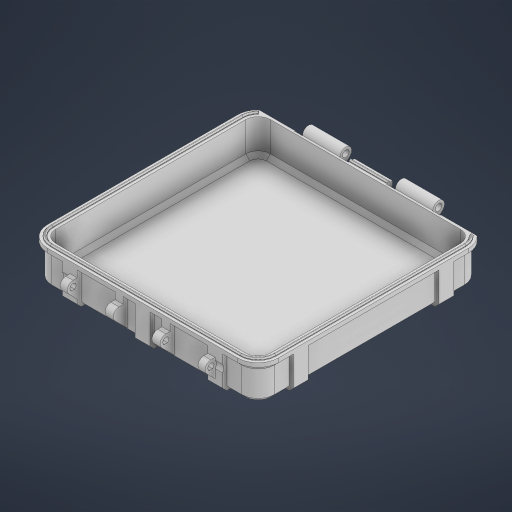
# Autodesk Inventor part: sumec_box-lid
Saved by Autodesk Inventor 2024 (Build 280153000, 153)
## iProperties
Created: 2024-03-05
Part Number: sumec_box-lid
Material: Všeobecné
Document SubType Name: Modeling
Designer: Simak
Density: 1 g/cm^3
Appearance: Výchozí
Author: Simak
Autodesk Inventor part; units mm, degrees
ref_plane "YZ Plane" through (0, 0, 0) normal (1, 0, 0) x (0, 1, 0)
ref_plane "XZ Plane" through (0, 0, 0) normal (0, 1, 0) x (-1, 0, 0)
sketch "velikost" plane through (0, 0, 0) normal (0, 1, 0) x (-1, 0, 0)
  line L0 (54.5, -54.5) -> (-54.5, -54.5)
  line L1 (-54.5, -54.5) -> (-54.5, 54.5)
  line L2 (-54.5, 54.5) -> (54.5, 54.5)
  line L3 (54.5, 54.5) -> (54.5, -54.5)
  line L4 (54.5, -54.5) -> (0, 0) construction
  line L5 (0, 0) -> (-54.5, -54.5) construction
  line L6 (0, 0) -> (-54.5, 54.5) construction
  dimension "d0" = 109
  dimension "d1" = 109
  constraints: 14 end point, 2 equal length, 2 parallel, 1 horizontal, 1 perpendicular
  measures "d0" distance of L0.start L0.end
  measures "d1" distance of L0.end L1.end
extrude "vyska" add sketch "velikost" along normal blind 18.5
fillet "Zaobleni_rohu" radius 8 4 edges at (-54.5, 9.25, 54.5) (54.5, 9.25, 54.5) (54.5, 9.25, -54.5) (-54.5, 9.25, -54.5)
shell "tloustka_sten" thickness 2 removed faces 1 at (15.5, 18.5, -12.8333)
sketch "vyztuhy-velikost" plane through (0, 18.5, 0) normal (0, 1, 0) x (1, 0, 0)
  arc A0 (-46.5, 52.5) -> (-52.5, 46.5) centre (-46.5, 46.5) ccw projected
  line L0 (-46.5, 52.5) -> (46.5, 52.5) projected
  arc A1 (52.5, 46.5) -> (46.5, 52.5) centre (46.5, 46.5) ccw projected
  line L1 (52.5, 46.5) -> (52.5, -46.5) projected
  arc A2 (46.5, -52.5) -> (52.5, -46.5) centre (46.5, -46.5) ccw projected
  line L2 (46.5, -52.5) -> (-46.5, -52.5) projected
  arc A3 (-52.5, -46.5) -> (-46.5, -52.5) centre (-46.5, -46.5) ccw projected
  line L3 (-52.5, -46.5) -> (-52.5, 46.5) projected
  arc A4 (-46.5, 54.5) -> (-54.5, 46.5) centre (-46.5, 46.5) ccw projected
  line L4 (-54.5, 46.5) -> (-54.5, -46.5) projected
  arc A5 (-54.5, -46.5) -> (-46.5, -54.5) centre (-46.5, -46.5) ccw projected
  line L5 (-46.5, -54.5) -> (46.5, -54.5) projected
  arc A6 (46.5, -54.5) -> (54.5, -46.5) centre (46.5, -46.5) ccw projected
  line L6 (54.5, -46.5) -> (54.5, 46.5) projected
  arc A7 (54.5, 46.5) -> (46.5, 54.5) centre (46.5, 46.5) ccw projected
  line L7 (46.5, 54.5) -> (-46.5, 54.5) projected
  line L8 (-39.2333, 54.5) -> (-39.2333, 56.5)
  line L9 (-39.2333, 56.5) -> (-31.9667, 56.5)
  line L10 (-31.9667, 56.5) -> (-31.9667, 54.5)
  line L11 (-3.6333, 54.5) -> (-3.6333, 56.5)
  line L12 (-3.6333, 56.5) -> (3.6333, 56.5)
  line L13 (3.6333, 56.5) -> (3.6333, 54.5)
  line L14 (31.9667, 54.5) -> (31.9667, 56.5)
  line L15 (31.9667, 56.5) -> (39.2333, 56.5)
  line L16 (39.2333, 56.5) -> (39.2333, 54.5)
  line L17 (46.5, 54.5) -> (-46.5, 54.5) projected
  line L18 (-3.6333, 56.5) -> (0, 54.5) construction
  line L19 (3.6333, 56.5) -> (0, 54.5) construction
  line L20 (-31.9667, 56.5) -> (-3.6333, 56.5) construction
  line L21 (3.6333, 56.5) -> (31.9667, 56.5) construction
  line L22 (-39.2333, 56.5) -> (-46.5, 56.5) construction
  line L23 (-46.5, 56.5) -> (-46.5, 54.5) construction
  line L24 (-52.5, 0) -> (52.5, 0)
  line L25 (0, 52.5) -> (0, -52.5)
  line L26 (46.5, -52.5) -> (-46.5, -52.5) projected
  line L27 (-54.5, -39.2333) -> (-56.5, -39.2333)
  line L28 (-56.5, -39.2333) -> (-56.5, -31.9667)
  line L29 (-56.5, -31.9667) -> (-54.5, -31.9667)
  line L30 (-54.5, 31.9667) -> (-56.5, 31.9667)
  line L31 (-56.5, 31.9667) -> (-56.5, 39.2333)
  line L32 (-56.5, 39.2333) -> (-54.5, 39.2333)
  line L33 (-56.5, -31.9667) -> (-56.5, 31.9667) construction
  line L34 (-56.5, -39.2333) -> (-56.5, -46.5) construction
  line L35 (-56.5, -46.5) -> (-54.5, -46.5) construction
  line L36 (-54.5, 46.5) -> (-54.5, -46.5) projected
  line L37 (-56.5, 39.2333) -> (-56.5, 46.5) construction
  line L38 (-56.5, 46.5) -> (-54.5, 46.5) construction
  line L39 (-54.5, 0) -> (-56.5, 31.9667) construction
  line L40 (-54.5, 0) -> (-56.5, -31.9667) construction
  line L41 (-39.2333, -54.5) -> (-39.2333, -56.5)
  line L42 (-39.2333, -56.5) -> (-31.9667, -56.5)
  line L43 (-31.9667, -56.5) -> (-31.9667, -54.5)
  line L44 (-3.6333, -54.5) -> (-3.6333, -56.5)
  line L45 (-3.6333, -56.5) -> (3.6333, -56.5)
  line L46 (3.6333, -56.5) -> (3.6333, -54.5)
  line L47 (31.9667, -54.5) -> (31.9667, -56.5)
  line L48 (31.9667, -56.5) -> (39.2333, -56.5)
  line L49 (39.2333, -56.5) -> (39.2333, -54.5)
  line L50 (46.5, -54.5) -> (-46.5, -54.5)
  line L51 (-3.6333, -56.5) -> (0, -54.5) construction
  line L52 (3.6333, -56.5) -> (0, -54.5) construction
  line L53 (-31.9667, -56.5) -> (-3.6333, -56.5) construction
  line L54 (3.6333, -56.5) -> (31.9667, -56.5) construction
  line L55 (-39.2333, -56.5) -> (-46.5, -56.5) construction
  line L56 (-46.5, -56.5) -> (-46.5, -54.5) construction
  line L57 (54.5, 46.5) -> (54.5, -46.5)
  line L58 (56.5, -31.9667) -> (56.5, 31.9667) construction
  line L59 (54.5, -39.2333) -> (56.5, -39.2333)
  line L60 (56.5, -39.2333) -> (56.5, -46.5) construction
  line L61 (56.5, -31.9667) -> (54.5, -31.9667)
  line L62 (56.5, -46.5) -> (54.5, -46.5) construction
  line L63 (56.5, -39.2333) -> (56.5, -31.9667)
  line L64 (56.5, 31.9667) -> (56.5, 39.2333)
  line L65 (56.5, 39.2333) -> (54.5, 39.2333)
  line L66 (54.5, 31.9667) -> (56.5, 31.9667)
  line L67 (54.5, 46.5) -> (54.5, -46.5)
  line L68 (56.5, 39.2333) -> (56.5, 46.5) construction
  line L69 (56.5, 46.5) -> (54.5, 46.5) construction
  line L70 (54.5, 0) -> (56.5, 31.9667) construction
  line L71 (54.5, 0) -> (56.5, -31.9667) construction
  point P0 (0, 0)
  point P1 (54.5, 39.2333)
  point P2 (54.5, 31.9667)
  point P3 (54.5, -31.9667)
  point P4 (39.2333, -54.5)
  point P5 (31.9667, -54.5)
  point P6 (3.6333, -54.5)
  point P7 (-3.6333, -54.5)
  point P8 (-31.9667, -54.5)
  point P9 (-39.2333, -54.5)
  point P10 (-54.5, -31.9667)
  point P11 (-54.5, 31.9667)
  point P12 (-54.5, 39.2333)
  dimension "d6" = 2
  dimension "d7" = 7.2667
  dimension "d8" = 2
  constraints: 120 end point, 25 symmetric about line, 20 point on line, 14 equal length, 11 perpendicular, 5 midpoint, 5 vertical, 2 horizontal, 5 other
  measures "d6" distance of L9.end L10.end
  measures "d7" distance of L11.end L12.end
  measures "d8" distance of L33.start L29.end
extrude "vyztuhy" add sketch "vyztuhy-velikost" against normal up to surface (18.5 mm away) contours L8 L9 L10 L7 | L4 L30 L31 L32 | L11 L12 L13 L7 | L4 L27 L28 L29 | L14 L15 L16 L7 | L5 L43 L42 L41 | L65 L64 L66 L6 | L5 L46 L45 L44 | L61 L63 L59 L6 | L5 L49 L48 L47
chamfer "Zkoseni_spodku" distance 2 angle 45 36 edges at (-17.8, 0, 54.5) (17.8, 0, 54.5) (0, 0, 56.5) (35.6, 0, 56.5) (42.8667, 0, 54.5) (52.1569, 0, 52.1569) (54.5, 0, 42.8667) (56.5, 0, 35.6) (54.5, 0, 0) (56.5, 0, -35.6) (52.1569, 0, -52.1569) (42.8667, 0, -54.5) (54.5, 0, -42.8667) (35.6, 0, -56.5) (17.8, 0, -54.5) (0, 0, -56.5) (-17.8, 0, -54.5) (-35.6, 0, -56.5) (-42.8667, 0, -54.5) (-52.1569, 0, -52.1569) (-54.5, 0, -42.8667) (-56.5, 0, -35.6) (-54.5, 0, 0) (-56.5, 0, 35.6) (-54.5, 0, 42.8667) (-52.1569, 0, 52.1569) (-42.8667, 0, 54.5) (-35.6, 0, 56.5) (-52.5, 2, 0) (-50.7426, 2, 50.7426) (0, 2, 52.5) (50.7426, 2, 50.7426) (52.5, 2, 0) (50.7426, 2, -50.7426) (0, 2, -52.5) (-50.7426, 2, -50.7426)
sketch "Náčrt4" plane through (39.2333, 18.5, -54.5) normal (1, 0, 0) x (0, 0, -1)
  line L0 (-2, 0) -> (-2, -14.5) projected
  line L1 (2, 0) -> (2, -16.5) projected
  line L2 (-8, 0) -> (0, 0) projected
  line L3 (-0.7, 0) -> (-0.7, 0.3)
  line L4 (-0.7, 0.3) -> (0.7, 0.3)
  line L5 (0.7, 0.3) -> (0.7, 0)
  line L6 (-0.7, 0.3) -> (-2, 0.3) construction
  line L7 (0.7, 0.3) -> (2, 0.3) construction
  line L8 (2, 0) -> (0, 0) projected
  line L9 (2, -4) -> (-2, -4)
  line L10 (-0.6, 0.3) -> (-0.1631, 0.9157)
  arc A0 (0.1631, 0.9157) -> (-0.1631, 0.9157) centre (0, 0.8) ccw
  line L11 (0.1631, 0.9157) -> (0.6, 0.3)
  point P0 (-54.5, -18.5)
  point P1 (0, 0.3)
  point P2 (0, 1)
  dimension "d16" = 1.4
  dimension "d71" = 4
  dimension "d72" = 0.3
  dimension "d75" = 1
  dimension "d76" = 0.2
  dimension "d77" = 0.6
  constraints: 16 end point, 9 point on line, 5 perpendicular, 3 point on circle, 3 vertical alignment, 2 equal length, 2 tangent, 1 centre point, 1 midpoint
  measures "d16" distance of L3.end L4.end
  measures "d71" distance between parallel lines of L9 L8
  measures "d72" distance between parallel lines of L8 L4
  measures "d75" distance from line of L8 point (0, 1)
  measures "d76" radius of A0
  measures "d77" horizontal distance of L11.end A0.centre
sketch "Náčrt3" plane through (0, 18.5, 0) normal (0, 1, 0) x (1, 0, 0)
  arc A0 (-46.5, 52.5) -> (-52.5, 46.5) centre (-46.5, 46.5) ccw projected
  line L0 (-46.5, 52.5) -> (46.5, 52.5) projected
  arc A1 (52.5, 46.5) -> (46.5, 52.5) centre (46.5, 46.5) ccw projected
  line L1 (52.5, 46.5) -> (52.5, -46.5) projected
  arc A2 (46.5, -52.5) -> (52.5, -46.5) centre (46.5, -46.5) ccw projected
  line L2 (46.5, -52.5) -> (-46.5, -52.5) projected
  arc A3 (-52.5, -46.5) -> (-46.5, -52.5) centre (-46.5, -46.5) ccw projected
  line L3 (-52.5, -46.5) -> (-52.5, 46.5) projected
  arc A4 (-46.5, 54.5) -> (-54.5, 46.5) centre (-46.5, 46.5) ccw projected
  line L4 (-54.5, 46.5) -> (-54.5, 39.2333) projected
  line L5 (-56.5, 31.9667) -> (-54.5, 31.9667) projected
  line L6 (-54.5, 31.9667) -> (-54.5, -31.9667) projected
  line L7 (-54.5, -31.9667) -> (-56.5, -31.9667) projected
  line L8 (-56.5, -31.9667) -> (-56.5, -39.2333) projected
  arc A5 (-54.5, -46.5) -> (-46.5, -54.5) centre (-46.5, -46.5) ccw projected
  line L9 (-46.5, -54.5) -> (-39.2333, -54.5) projected
  line L10 (-39.2333, -54.5) -> (-39.2333, -56.5) projected
  line L11 (-39.2333, -56.5) -> (-31.9667, -56.5) projected
  line L12 (-31.9667, -56.5) -> (-31.9667, -54.5) projected
  line L13 (-31.9667, -54.5) -> (-3.6333, -54.5) projected
  line L14 (-3.6333, -54.5) -> (-3.6333, -56.5) projected
  line L15 (-3.6333, -56.5) -> (3.6333, -56.5) projected
  line L16 (3.6333, -56.5) -> (3.6333, -54.5) projected
  line L17 (3.6333, -54.5) -> (31.9667, -54.5) projected
  line L18 (31.9667, -54.5) -> (31.9667, -56.5) projected
  line L19 (31.9667, -56.5) -> (39.2333, -56.5) projected
  line L20 (39.2333, -56.5) -> (39.2333, -54.5) projected
  line L21 (39.2333, -54.5) -> (46.5, -54.5) projected
  arc A6 (46.5, -54.5) -> (54.5, -46.5) centre (46.5, -46.5) ccw projected
  line L22 (54.5, -46.5) -> (54.5, -39.2333) projected
  line L23 (56.5, -31.9667) -> (54.5, -31.9667) projected
  line L24 (54.5, -31.9667) -> (54.5, 31.9667) projected
  line L25 (54.5, 31.9667) -> (56.5, 31.9667) projected
  line L26 (56.5, 31.9667) -> (56.5, 39.2333) projected
  arc A7 (54.5, 46.5) -> (46.5, 54.5) centre (46.5, 46.5) ccw projected
  line L27 (46.5, 54.5) -> (39.2333, 54.5) projected
  line L28 (39.2333, 54.5) -> (39.2333, 56.5) projected
  line L29 (39.2333, 56.5) -> (31.9667, 56.5) projected
  line L30 (31.9667, 56.5) -> (31.9667, 54.5) projected
  line L31 (31.9667, 54.5) -> (3.6333, 54.5) projected
  line L32 (3.6333, 54.5) -> (3.6333, 56.5) projected
  line L33 (3.6333, 56.5) -> (-3.6333, 56.5) projected
  line L34 (-3.6333, 56.5) -> (-3.6333, 54.5) projected
  line L35 (-3.6333, 54.5) -> (-31.9667, 54.5) projected
  line L36 (-31.9667, 54.5) -> (-31.9667, 56.5) projected
  line L37 (-31.9667, 56.5) -> (-39.2333, 56.5) projected
  line L38 (-39.2333, 56.5) -> (-39.2333, 54.5) projected
  line L39 (-39.2333, 54.5) -> (-46.5, 54.5) projected
  line L40 (-54.5, 39.2333) -> (-56.5, 39.2333) projected
  line L41 (-56.5, 39.2333) -> (-56.5, 31.9667) projected
  line L42 (-56.5, -39.2333) -> (-54.5, -39.2333) projected
  line L43 (-54.5, -39.2333) -> (-54.5, -46.5) projected
  line L44 (54.5, -39.2333) -> (56.5, -39.2333) projected
  line L45 (56.5, -39.2333) -> (56.5, -31.9667) projected
  line L46 (56.5, 39.2333) -> (54.5, 39.2333) projected
  line L47 (54.5, 39.2333) -> (54.5, 46.5) projected
  point P0 (0, 0)
sweep "tesnici_drazka" add profiles "Náčrt4" path "Náčrt3" path curves L0 A0 L3 A3 L2 A2 L1 A1
chamfer "tesnici_drazka-zkoseni" distance 2 angle 45 18 edges at (53.5711, 14.5, -53.5711) (42.8667, 14.5, -56.5) (56.5, 14.5, -42.8667) (17.8, 14.5, -56.5) (-17.8, 14.5, -56.5) (56.5, 14.5, 0) (56.5, 14.5, 42.8667) (53.5711, 14.5, 53.5711) (42.8667, 14.5, 56.5) (-53.5711, 14.5, -53.5711) (-56.5, 14.5, -42.8667) (-42.8667, 14.5, -56.5) (-56.5, 14.5, 0) (-53.5711, 14.5, 53.5711) (-42.8667, 14.5, 56.5) (-56.5, 14.5, 42.8667) (17.8, 14.5, 56.5) (-17.8, 14.5, 56.5)
sketch "Náčrt16" plane through (31.9667, 0, -54.5) normal (-1, 0, 0) x (0, 0, 1)
  line L0 (-2, 16.5) -> (-2, 2) projected
  line L1 (0, 0) -> (-2, 2) projected
  line L2 (2, 0) -> (0, 0) projected
  line L3 (0, 2) -> (2, 0) projected
  line L4 (0, 14.5) -> (0, 2) projected
  line L5 (-2, 16.5) -> (0, 14.5) projected
  line L6 (8, 18.5) -> (-2, 18.5) projected
  circle A0 centre (-2, 18.5) radius 1.65
  circle A1 centre (-2, 18.5) radius 2.7
  circle A2 centre (-2, 18.5) radius 2.875
  circle A3 centre (-2, 18.5) radius 3.025
  line L7 (0, 12.4341) -> (-4.0329, 16.4671)
  point P0 (54.5, 0)
  point P1 (0.875, 18.5)
  point P2 (-1.1092, 15.6092)
  point P3 (1.025, 18.5)
  point P4 (-3.3677, 15.8019)
  point P5 (-2, 14.4341)
  point P6 (-2, 15.475)
  dimension "d148" = 5.75
  dimension "d147" = 3.3
  dimension "d149" = 5.4
  dimension "d150" = 0.15
  dimension "d151" = 45
  constraints: 3 centre point, 3 coincident, 2 end point, 1 point on line, 4 other
  measures "d147" diameter of A0
  measures "d149" diameter of A1
  measures "d151" angle of L4 L7
extrude "Vysunutí23" cut sketch "Náčrt16" along normal blind 22.65 and the other way blind 3.65 contours L5 A1 L0 | L0 A1 L5 | A1 L5 A2 L0 | L0 A2 L6 A1 | A1 L6 A2 L5 | A2 L5 A3 L0 | L0 A3 L7 A2 | A2 L6 A3 L5 | L7 A3 L6 A2 | A0
extrude "Vysunutí24" cut sketch "Náčrt16" against normal through all contours L5 A1 L0 | L0 A1 L5 | A0
extrude "Vysunutí25" add sketch "Náčrt16" along normal blind 18.4 contours L5 A1 L0 | L0 A1 L5 | A1 L5 A2 L0 | L0 A2 L6 A1 | A1 L6 A2 L5 | A2 L5 A3 L0 | L0 A3 L7 A2 | A2 L6 A3 L5 | A3 L5 L4 L7 L0 | L0 L7 A3
extrude "Vysunutí26" cut sketch "Náčrt16" along normal blind 0.1 contours L5 A1 L0 | L0 A1 L5 | A1 L5 A2 L0 | L0 A2 L6 A1 | A1 L6 A2 L5 | A2 L5 A3 L0 | L0 A3 L7 A2 | A2 L6 A3 L5 | L0 L7 A3 | L7 A3 L6 A2 | A0
sketch "Náčrt17" plane through (0, 18.5, 0) normal (0, 1, 0) x (1, 0, 0)
  arc A0 (-46.5, 52.5) -> (-52.5, 46.5) centre (-46.5, 46.5) ccw projected
  line L0 (-46.5, 52.5) -> (46.5, 52.5) projected
  arc A1 (52.5, 46.5) -> (46.5, 52.5) centre (46.5, 46.5) ccw projected
  line L1 (52.5, 46.5) -> (52.5, -46.5) projected
  arc A2 (46.5, -52.5) -> (52.5, -46.5) centre (46.5, -46.5) ccw projected
  line L2 (46.5, -52.5) -> (-46.5, -52.5) projected
  arc A3 (-52.5, -46.5) -> (-46.5, -52.5) centre (-46.5, -46.5) ccw projected
  line L3 (-52.5, -46.5) -> (-52.5, 46.5) projected
  arc A4 (-46.5, 53.8) -> (-53.8, 46.5) centre (-46.5, 46.5) ccw projected
  line L4 (-53.8, 46.5) -> (-53.8, -46.5) projected
  arc A5 (-53.8, -46.5) -> (-46.5, -53.8) centre (-46.5, -46.5) ccw projected
  line L5 (-46.5, -53.8) -> (46.5, -53.8) projected
  arc A6 (46.5, -53.8) -> (53.8, -46.5) centre (46.5, -46.5) ccw projected
  line L6 (53.8, -46.5) -> (53.8, 46.5) projected
  arc A7 (53.8, 46.5) -> (46.5, 53.8) centre (46.5, 46.5) ccw projected
  line L7 (46.5, 53.8) -> (35.6167, 53.8) projected
  line L8 (35.6167, 53.8) -> (35.6167, 53.475) projected
  line L9 (35.6167, 53.475) -> (31.8667, 53.475) projected
  line L10 (31.8667, 53.475) -> (31.8667, 53.625) projected
  line L11 (31.8667, 53.625) -> (13.5667, 53.625) projected
  line L12 (13.5667, 53.475) -> (13.5667, 53.625) projected
  line L13 (13.5667, 53.475) -> (9.3167, 53.475) projected
  line L14 (9.3167, 53.475) -> (9.3167, 53.8) projected
  line L15 (9.3167, 53.8) -> (-46.5, 53.8) projected
  arc A8 (-46.5, 56.5) -> (-56.5, 46.5) centre (-46.5, 46.5) ccw projected
  line L16 (-56.5, 46.5) -> (-56.5, -46.5) projected
  arc A9 (-56.5, -46.5) -> (-46.5, -56.5) centre (-46.5, -46.5) ccw projected
  line L17 (-46.5, -56.5) -> (46.5, -56.5) projected
  arc A10 (46.5, -56.5) -> (56.5, -46.5) centre (46.5, -46.5) ccw projected
  line L18 (56.5, -46.5) -> (56.5, 46.5) projected
  arc A11 (56.5, 46.5) -> (53.3345, 53.8) centre (46.5, 46.5) ccw projected
  line L19 (53.3345, 53.8) -> (51.2329, 53.8) projected
  arc A12 (55.2, 46.5) -> (51.2329, 53.8) centre (46.5, 46.5) ccw projected
  line L20 (55.2, -46.5) -> (55.2, 46.5) projected
  arc A13 (46.5, -55.2) -> (55.2, -46.5) centre (46.5, -46.5) ccw projected
  line L21 (-46.5, -55.2) -> (46.5, -55.2) projected
  arc A14 (-55.2, -46.5) -> (-46.5, -55.2) centre (-46.5, -46.5) ccw projected
  line L22 (-55.2, 46.5) -> (-55.2, -46.5) projected
  arc A15 (-46.5, 55.2) -> (-55.2, 46.5) centre (-46.5, 46.5) ccw projected
  spline S0 degree 8 poles (46.5, 55.8737) (47.0163, 55.8737) (47.5323, 55.8475) (48.0473, 55.7951) (48.5603, 55.7176) (49.0703, 55.6177) (49.5764, 55.4985) (50.0774, 55.3641) (50.7861, 55.1565) (50.9987, 55.092) (51.21, 55.0258) (51.4199, 54.9585) (51.6283, 54.8905) (51.8351, 54.8221) (52.0401, 54.7539) (52.2432, 54.6863) knots 0 0 0 0 0 0 0 0 0 0.698385 0.698385 0.698385 0.698385 0.698385 0.698385 0.698385 1 1 1 1 1 1 1 1 1 projected
  line L23 (39.2333, 55.8737) -> (46.5, 55.8737) projected
  line L24 (39.2333, 56.5) -> (39.2333, 55.8737) projected
  line L25 (35.6167, 56.5) -> (39.2333, 56.5) projected
  line L26 (35.6167, 53.8) -> (35.6167, 56.5) projected
  line L27 (46.5, 53.8) -> (35.6167, 53.8) projected
  line L28 (35.6167, 53.8167) -> (35.6167, 53.8) projected
  line L29 (47.6071, 53.8167) -> (35.6167, 53.8167) projected
  line L30 (51.207, 53.8167) -> (51.0195, 53.8167) projected
  line L31 (53.3345, 53.8) -> (51.2329, 53.8) projected
  spline S1 degree 6 poles (52.2432, 54.6863) (52.3272, 54.6273) (52.4089, 54.5685) (52.4878, 54.5102) (52.5637, 54.4527) (52.6363, 54.3964) (52.7493, 54.307) (52.7917, 54.273) (52.8326, 54.2397) (52.8719, 54.2073) (52.9096, 54.1759) (52.9724, 54.1229) (52.9985, 54.1008) (53.0235, 54.0793) (53.0475, 54.0586) (53.0703, 54.0387) (53.1714, 53.9501) (53.2361, 53.8916) (53.2852, 53.8462) (53.318, 53.8154) (53.3345, 53.8) (53.3345, 53.8) knots 0 0 0 0 0 0 0 0.258993 0.258993 0.258993 0.258993 0.258993 0.423699 0.423699 0.423699 0.423699 0.423699 0.547895 0.547895 0.547895 0.547895 0.547895 1 1 1 1 1 1 1 projected
  line L32 (35.6167, 53.475) -> (35.6167, 52.5)
  line L33 (46.5, 46.5) -> (52.5, 52.8)
  line L34 (9.3167, 55.2) -> (-46.5, 55.2) projected
  line L35 (9.3167, 55.2) -> (9.3167, 56.5) projected
  line L36 (9.3167, 56.5) -> (-46.5, 56.5) projected
  point P0 (0, 0)
  point P1 (51.5345, 51.7862)
  point P2 (46.7329, 24.3)
  point P3 (51.2329, 53.8)
  point P4 (53.3345, 53.8)
  point P5 (51.7329, 54.3)
  dimension "d162" = 1
  constraints: 4 end point, 1 horizontal alignment, 1 perpendicular, 1 point on circle, 1 point on line, 5 other
  measures "d162" distance from line of L19 L33.end
extrude "Vysunutí27" cut sketch "Náčrt17" along normal through all contours L26 L25 L24 L23 S0 S1 L19 A12 L33 A7 L7
sketch "Náčrt18" plane through (31.8667, 0, -54.5) normal (1, 0, 0) x (0, 0, -1)
  line L0 (4.0329, 16.4671) -> (2, 14.4341) projected
  arc A0 (4.0329, 16.4671) -> (-0.875, 18.5) centre (2, 18.5) ccw projected
  line L1 (-1.025, 18.5) -> (-0.875, 18.5) projected
  arc A1 (-1.025, 18.5) -> (2, 15.475) centre (2, 18.5) ccw projected
  line L2 (2, 14.4341) -> (2, 15.475) projected
  circle A2 centre (2, 18.5) radius 1.65 projected
  circle A3 centre (2, 18.5) radius 2.875
  line L3 (-0.139, 16.361) -> (2, 14.222)
  line L4 (2, 16.5) -> (2, 2) projected
  arc A4 (-1.025, 18.5) -> (1.1092, 15.6092) centre (2, 18.5) ccw projected
  point P0 (-54.5, 0)
  point P1 (-0.139, 16.361)
  dimension "d165" = 45
  constraints: 3 point on circle, 2 end point, 1 coincident, 1 horizontal alignment, 1 point on line, 1 tangent, 2 other
  measures "d165" angle of L4 L3
extrude "Vysunutí28" cut sketch "Náčrt18" along normal up to surface (3.75 mm away) contours L4 L3 A1 L2
sketch "Náčrt19" plane through (13.5667, 0, -54.5) normal (-1, 0, 0) x (0, 0, 1)
  line L0 (-4.0329, 16.4671) -> (-1.8939, 14.3281) projected
  arc A0 (0.875, 18.5) -> (-4.0329, 16.4671) centre (-2, 18.5) ccw projected
  line L1 (1.025, 18.5) -> (0.875, 18.5) projected
  arc A1 (0.139, 16.361) -> (1.025, 18.5) centre (-2, 18.5) ccw projected
  line L2 (0.139, 16.361) -> (-1.8939, 14.3281) projected
  circle A2 centre (-2, 18.5) radius 1.65 projected
  point P0 (54.5, 0)
extrude "Vysunutí29" cut sketch "Náčrt19" along normal up to surface (4.25 mm away)
mirror "Zrcadlit4" about plane through (0, 0, 0) normal (1, 0, 0) of "Vysunutí23", "Vysunutí24", "Vysunutí25", "Vysunutí26", "Vysunutí27", "Vysunutí28", "Vysunutí29"
sketch "latch-main_nacrt" plane through (31.9667, 0, 52.5) normal (-1, 0, 0) x (0, 0, 1)
  line L0 (4, 16.5) -> (4, 2) projected
  line L1 (2, 0) -> (4, 2) projected
  line L2 (0, 0) -> (2, 0) projected
  line L3 (2, 2) -> (0, 0) projected
  line L4 (2, 14.5) -> (2, 2) projected
  line L5 (4, 16.5) -> (2, 14.5) projected
  line L6 (4, 18.5) -> (-6, 18.5) projected
  line L7 (2.7, 18.8) -> (-6, 18.8) projected
  line L8 (1.25, 23) -> (1.25, 25) projected
  line L9 (2.7, 18.8) -> (2.7, 18.5) projected
  line L10 (4, 18.5) -> (4, 16.5) projected
  circle A0 centre (6.05, 10.3) radius 1.55
  line L11 (5.3, 8.9435) -> (5.3, 9.1)
  line L12 (5.3, 9.1) -> (6.8, 9.1)
  line L13 (6.8, 9.1) -> (6.8, 8.9435)
  circle A1 centre (6.05, 10.3) radius 2.875
  line L14 (6.05, 13.175) -> (2, 13.175)
  line L15 (2, 2.1841) -> (8.0829, 8.2671)
  circle A2 centre (6.05, 10.3) radius 2.7
  point P0 (-52.5, 0)
  point P1 (4, 12.3157)
  point P2 (4, 8.2843)
  dimension "d52" = 3.1
  dimension "d53" = 8.2
  dimension "d54" = 4.05
  dimension "d55" = 2.75
  dimension "d56" = 1.5
  dimension "d57" = 5.75
  dimension "d58" = 45
  dimension "d63" = 5.4
  constraints: 10 end point, 4 point on circle, 3 centre point, 3 perpendicular, 2 coincident, 2 point on line, 2 tangent, 1 parallel, 1 vertical, 2 other
  measures "d52" diameter of A0
  measures "d54" distance from line of L4 A0.centre
  measures "d56" distance of L11.end L12.end
  measures "d57" diameter of A1
  measures "d58" angle of L4 L15
  measures "d63" diameter of A2
extrude "Vysunutí14" cut sketch "latch-main_nacrt" against normal up to next contours A2 L0 | L0 A2
extrude "Vysunutí12" add sketch "latch-main_nacrt" against normal blind 3.5 contours L14 A1 L0 | L0 A1 L15 L4 L14 | A1 L0 A2 | L0 A2 A1 | A2 L0 | L0 A2 | A1 L15 L0 | L11 L12 L13 A0 picked at (5.9979, 8.986)
ref_plane "Pracovní rovina3" through (13.4667, 0, 52.5) normal (-1, 0, 0) x (0, 0, 1)
sketch "Náčrt10" plane through (13.4667, 0, 52.5) normal (-1, 0, 0) x (0, 0, 1)
  arc A0 (6.8, 8.9435) -> (5.3, 8.9435) centre (6.05, 10.3) ccw projected
  line L0 (6.8, 8.9435) -> (6.8, 9.1) projected
  line L1 (6.8, 9.1) -> (5.3, 9.1) projected
  line L2 (5.3, 9.1) -> (5.3, 8.9435) projected
  line L3 (4, 4.1841) -> (8.0829, 8.2671) projected
  arc A1 (8.0829, 8.2671) -> (6.05, 13.175) centre (6.05, 10.3) ccw projected
  line L4 (6.05, 13.175) -> (4, 13.175) projected
  line L5 (4, 16.5) -> (4, 13.175) projected
  line L6 (2, 14.5) -> (4, 16.5) projected
  line L7 (2, 2) -> (2, 14.5) projected
  line L8 (0, 0) -> (2, 2) projected
  line L9 (2, 0) -> (0, 0) projected
  line L10 (4, 2) -> (2, 0) projected
  line L11 (4, 4.1841) -> (4, 2) projected
  line L12 (4, 13.175) -> (2, 13.175)
  line L13 (4, 4.1841) -> (2, 2.1841)
  line L14 (4, 13.175) -> (2, 14.5)
  point P0 (-52.5, 0)
  constraints: 6 end point, 2 collinear, 2 point on line
extrude "Vysunutí15" add sketch "Náčrt10" along normal blind 4 contours L13 L7 L12 L4 A1 L3 | L7 L14 L12 | L14 L6 L5
sketch "Náčrt12" plane through (9.4667, 0, 52.5) normal (-1, 0, 0) x (0, 0, 1)
  line L0 (2, 2.1841) -> (8.0829, 8.2671) projected
  arc A0 (8.0829, 8.2671) -> (6.05, 13.175) centre (6.05, 10.3) ccw projected
  line L1 (6.05, 13.175) -> (4, 13.175) projected
  line L2 (6.8, 9.1) -> (5.3, 9.1) projected
  line L3 (5.3, 9.1) -> (5.3, 8.9435) projected
  arc A1 (6.8, 8.9435) -> (5.3, 8.9435) centre (6.05, 10.3) ccw projected
  line L4 (6.8, 8.9435) -> (6.8, 9.1) projected
  line L5 (4, 13.175) -> (4, 16.5) projected
  line L6 (2, 14.5) -> (4, 16.5) projected
  line L7 (2, 2.1841) -> (2, 14.5) projected
  point P0 (-52.5, 0)
extrude "Vysunutí16" add sketch "Náčrt12" against normal blind 0.5 contours L2 L3 A1 L4
mirror "latch-zrcadleni" about plane through (0, 0, 0) normal (1, 0, 0) of "Vysunutí16", "Vysunutí14", "Vysunutí12", "Vysunutí15"
fillet "Zaoblení2" radius 1 8 edges at (-42.8667, 15.8736, -55.8737) (-49.4352, 15.9845, -55.519) (-53.0393, 17.3323, -54.0656) (-37.425, 15.8, -56.5) (37.425, 15.8, -56.5) (49.4352, 15.9845, -55.519) (42.8667, 15.8736, -55.8737) (53.0393, 17.3323, -54.0656)
ref_plane "Pracovní rovina4" through (-13.4667, 0, 52.5) normal (-1, 0, 0) x (0, 0, 1)
